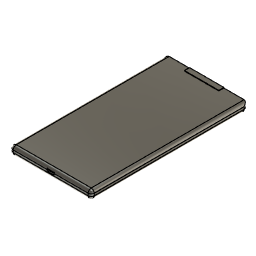
phone v1 (Autodesk Fusion 360 design; units mm, degrees)
Autodesk Fusion 360 part; units mm, degrees
sketch "Sketch1" plane through (0, 0, 0) normal (0, 0, 1) x (1, 0, 0)
  line L0 (0, 0) -> (80, 0)
  line L1 (80, 0) -> (80, 154)
  line L2 (80, 154) -> (0, 154)
  line L3 (0, 154) -> (0, 0)
  line L4 (40, 154) -> (40, 0) construction
  line L5 (80, 75) -> (0, 75) construction
  line L6 (40, 149) -> (57, 149)
  line L7 (40, 149) -> (23, 149)
  line L8 (23, 149) -> (23, 154)
  line L9 (57, 149) -> (57, 154)
  line L10 (0, 154, 0) -> (0, 154, 8.27)
  line L11 (0, 154, 8.27) -> (0, 0, 8.27)
  line L12 (0, 0, 8.27) -> (0, 0, 0)
  line L13 (80, 0, 0) -> (80, 0, 8.27)
  line L14 (80, 0, 8.27) -> (80, 154, 8.27)
  line L15 (80, 154, 8.27) -> (80, 154, 0)
  line L16 (0, 0, 8.27) -> (80, 0, 8.27)
  line L17 (80, 154, 8.27) -> (0, 154, 8.27)
  line L18 (74.5391, 150.0536, 8.27) -> (74.5391, 126.0536, 8.27)
  line L19 (74.5391, 126.0536, 8.27) -> (62.5391, 126.0536, 8.27)
  line L20 (62.5391, 126.0536, 8.27) -> (62.5391, 150.0536, 8.27)
  circle A0 centre (68, 143) radius 4.5
  circle A1 centre (68, 132) radius 4.5
  line L21 (0, 142, 2) -> (0, 142, 3)
  line L22 (0, 142, 3) -> (0, 136.6, 3)
  line L23 (0, 136.6, 3) -> (0, 136.6, 2)
  line L24 (0, 136.6, 2) -> (0, 142, 2)
  line L25 (0, 136.6, 3) -> (0, 136.6, 1)
  line L26 (0, 136.6, 1) -> (0, 142, 1)
  line L27 (0, 142, 1) -> (0, 142, 3)
  line L28 (0, 133.5, 3) -> (0, 117.5, 3)
  line L29 (0, 117.5, 3) -> (0, 117.5, 3.0422)
  line L30 (0, 117.5, 3.0422) -> (0, 133.5, 3.0422)
  line L31 (0, 133.5, 3.0422) -> (0, 133.5, 3)
  line L32 (0, 117.5, 3) -> (0, 117.5, 1.5)
  line L33 (0, 117.5, 1.5) -> (0, 133.5, 1.5)
  line L34 (0, 133.5, 1.5) -> (0, 133.5, 3)
  line L35 (0, 116, 3) -> (0, 100, 3)
  line L36 (0, 100, 3) -> (0, 100, 1.5)
  line L37 (0, 100, 1.5) -> (0, 116, 1.5)
  line L38 (0, 116, 1.5) -> (0, 116, 3)
  line L39 (74.5391, 150.0536, 8.27) -> (62.5391, 150.0536, 8.27)
  line L40 (80, 0, 4) -> (0, 0, 4) construction
  line L41 (40, 0, 4) -> (36.5, 0, 4)
  line L42 (40, 0, 4) -> (43.5, 0, 4)
  line L43 (43.5, 0, 4) -> (43.5, 0, 6.25)
  line L44 (43.5, 0, 6.25) -> (36.5, 0, 6.25)
  line L45 (36.5, 0, 6.25) -> (36.5, 0, 4)
  dimension "d15" = 80
  dimension "d16" = 154
  dimension "d17" = 5
  dimension "d18" = 17
  dimension "d19" = 17
  dimension "d20" = 8.27
  dimension "d21" = 154
  dimension "d22" = 8.27
  dimension "d23" = 8.27
  dimension "d24" = 154
  dimension "d25" = 8.27
  dimension "d26" = 24
  dimension "d27" = 12
  dimension "d28" = 24
  dimension "d29" = 9
  dimension "d30" = 9
  dimension "d31" = 1
  dimension "d32" = 5.4
  dimension "d33" = 1
  dimension "d34" = 2
  dimension "d35" = 5.4
  dimension "d36" = 16
  dimension "d37" = 0.0422
  dimension "d38" = 1.5
  dimension "d39" = 16
  dimension "d40" = 16
  dimension "d41" = 1.5
  dimension "d42" = 16
  dimension "d63" = 3.5
  dimension "d64" = 3.5
  dimension "d65" = 2.25
  dimension "d66" = 7
  dimension "d67" = 2.25
  constraint horizontal L0
  constraint vertical L1
  constraint horizontal L2
  constraint vertical L3
  constraint coincident L0.start L3.end
  constraint midpoint L2 L4.start
  constraint midpoint L0 L4.end
  constraint coincident L1 L5.start
  constraint coincident L3 L5.end
  constraint perpendicular L3 L5
  constraint coincident L4 L6.start
  constraint perpendicular L4 L7
  constraint coincident L2 L8.end
  constraint perpendicular L2 L8
  constraint coincident L2 L9.end
  constraint perpendicular L2 L9
  measures "d15" distance of L0.start L0.end
  measures "d16" distance of L0.start L2.end
  measures "d17" distance of L4.start L6.start
  measures "d18" distance of L6.start L6.end
  measures "d19" distance of L6.start L7.end
  measures "d20" distance of L2.end L3.start
  measures "d21" distance of L2.end L0.start
  measures "d22" distance of L0.start L3.end
  measures "d23" distance of L0.end L1.start
  measures "d24" distance of L0.end L1.end
  measures "d25" distance of L1.end L2.start
  measures "d29" diameter of A0
  measures "d30" diameter of A1
extrude "Extrude10" add sketch "Sketch1" along normal blind 1.3 contours L41 L42 L43 L44 L45 in plane through (0, 0, 0) normal (0, 1, 0) makes body 1
extrude "Extrude3" add sketch "Sketch1" against normal blind 9.07 separate body contours L18 L19 L20 L39 in plane through (0, 0, 8.27) normal (0, 0, 1) makes body 2
extrude "Extrude1" add sketch "Sketch1" along normal blind 1.3 separate body contours L21 L22 L23 L24 L25 L27 | L28 L32 L33 L34 | L35 L36 L37 L38 in plane through (0, 0, 0) normal (1, 0, 0) makes body 3 at (0, 105.3333, 2) makes body 4 at (0, 122.8333, 2.5) makes body 5 at (0.4333, 138.4, 2)
extrude "Extrude2" add sketch "Sketch1" against normal blind 1.3 separate body contours A0 | A1 makes body 6 at (67.6662, 144.4624, 0) makes body 7 at (67.8879, 133.429, 0)
extrude "Extrude4" add sketch "Sketch1" along normal blind 8.77 separate body contours L2 L6 L7 L8 L9 makes body 8
extrude "Extrude5" add sketch "Sketch1" along normal blind 8.27 contours L0 L1 L2 L3 L6 L7 L8 L9 bodies 2 3 4 5 6 7 8
extrude "Extrude6" add sketch "Sketch1" along normal blind 1.3 contours L21 L22 L23 L24 L25 L27 | L28 L32 L33 L34 | L35 L36 L37 L38 in plane through (0, 0, 0) normal (1, 0, 0) bodies 2
extrude "Extrude7" add sketch "Sketch1" along normal blind 1 contours L21 L22 L23 L24 L25 L27 | L28 L32 L33 L34 | L35 L36 L37 L38 in plane through (0, 0, 0) normal (1, 0, 0) bodies 2
extrude "Extrude9" add sketch "Sketch1" against normal blind 1.3 separate body contours L21 L22 L23 L24 L25 L27 | L28 L32 L33 L34 | L35 L36 L37 L38 in plane through (0, 0, 0) normal (1, 0, 0) makes body 9 at (0, 105.3333, 2) makes body 10 at (0, 122.8333, 2.5) makes body 11 at (-0.4333, 138.4, 2)
fillet "Fillet1" radius 3 15 edges at (0, 0, 4.135) (80, 0, 4.135) (40, 0, 8.27) (40, 0, 0) (80, 77, 8.27) (80, 77, 0) (80, 154, 4.135) (40, 154, 0) (0, 154, 4.135) (0, 77, 8.27) (0, 77, 0) (74.5391, 138.0536, -0.8) (68.5391, 150.0536, -0.8) (62.5391, 138.0536, -0.8) (68.5391, 126.0536, -0.8) on bodies 2
equation "totalwidth = 80 mm"
equation "totallength = 154 mm"
equation "notchwidth = 34 mm"
equation "notchheight = 5 mm"
equation "camerabulge = 1.3 mm"
equation "cameraheight = 24 mm"
equation "camerawidth = 12 mm"
equation "volumebuttonwidth = 3 mm"
equation "volumebuttonheight = 16 mm"
equation "ringerwidth = 1 mm"
equation "ringerhousing = 2 mm"
equation "ringerheight = 5.4 mm"
equation "totalphoneheight = 8.27 mm"
equation "radius = totalphoneheight / 2"
equation "d15 = totalwidth"
equation "d16 = totallength"
equation "d17 = notchheight"
equation "d18 = notchwidth / 2"
equation "d19 = notchwidth / 2"
equation "d20 = totalphoneheight"
equation "d21 = totallength"
equation "d22 = totalphoneheight"
equation "d23 = totalphoneheight"
equation "d24 = totallength"
equation "d25 = totalphoneheight"
equation "d26 = cameraheight"
equation "d27 = camerawidth"
equation "d28 = cameraheight"
equation "d31 = ringerwidth"
equation "d32 = ringerheight"
equation "d33 = ringerwidth"
equation "d34 = ringerhousing"
equation "d35 = ringerheight"
equation "d36 = volumebuttonheight"
equation "d38 = volumebuttonwidth / 2"
equation "d39 = volumebuttonheight"
equation "d40 = volumebuttonheight"
equation "d41 = volumebuttonwidth / 2"
equation "d42 = volumebuttonheight"
equation "d43 = camerabulge"
equation "d45 = -camerabulge"
equation "d47 = -totalphoneheight - camerabulge + 0.5 mm"
equation "d49 = totalphoneheight + 0.5 mm"
equation "d51 = totalphoneheight"
equation "d53 = camerabulge"
equation "d59 = -camerabulge"
equation "portwidth = 7 mm"
equation "portheight = 2.25 mm"
equation "d63 = portwidth / 2"
equation "d64 = portwidth / 2"
equation "d65 = portheight"
equation "d66 = portwidth"
equation "d67 = portheight"
equation "d68 = -camerabulge"
